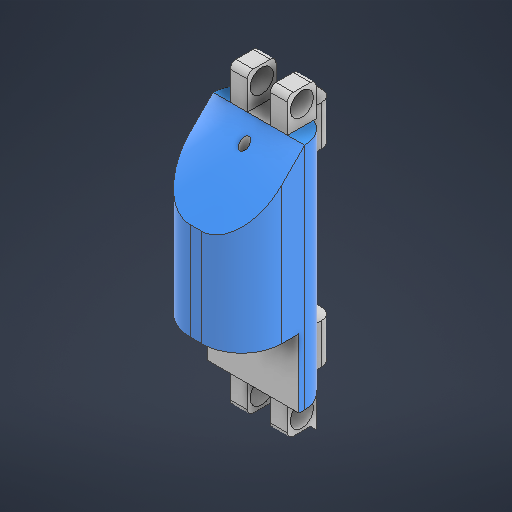
# Autodesk Inventor part: FingerBase
Saved by Autodesk Inventor 2026 (Build 300175050, 175E)
## iProperties
Created: 2026-05-23
Part Number: FingerBase
Material: Generic
Document SubType Name: Modeling
Designer: SaiAn
Density: 1 g/cm^3
Appearance: Default
Author: SaiAn
Autodesk Inventor part; units mm, degrees
ref_plane "YZ Plane" through (0, 0, 0) normal (1, 0, 0) x (0, 1, 0)
ref_plane "XZ Plane" through (0, 0, 0) normal (0, 1, 0) x (-1, 0, 0)
ref_plane "XY Plane" through (0, 0, 0) normal (0, 0, 1) x (1, 0, 0)
sketch "Sketch2" plane through (0, 0, 0) normal (0, 0, 1) x (1, 0, 0)
  line L0 (0, 0) -> (16, 0)
  line L1 (16, 0) -> (16, 40)
  line L2 (16, 40) -> (0, 40)
  line L3 (0, 40) -> (0, 0)
  dimension "d0" = 16
  dimension "d1" = 40
  constraints: 8 end point, 2 parallel, 1 horizontal, 1 perpendicular
  measures "d0" distance of L2.end L1.end
  measures "d1" distance of L1.end L0.end
extrude "Extrusion1" add sketch "Sketch2" along normal blind 16
fillet "Fillet1" radius 7 2 edges at (16, 20, 16) (0, 20, 16)
fillet "Fillet2" radius 5 2 edges at (16, 20, 0) (0, 20, 0)
sketch "Sketch3" plane through (16, 0, 9) normal (1, 0, 0) x (0, 0, -1)
  line L0 (4, 0) -> (4, 40) projected
  line L1 (4, 40) -> (-7, 29)
  line L2 (-7, 0) -> (-7, 40) projected
  line L3 (4, 40) -> (19.5563, 40) construction
  line L4 (-7, 29) -> (-7, 40)
  line L5 (-7, 40) -> (4, 40)
  line L6 (1, 0) -> (12.3137, 0) construction
  line L7 (-7, 8) -> (-7, 0)
  line L8 (1, 0) -> (19.9296, 0) construction
  line L9 (-7, 17.1561) -> (-7, 8)
  point P0 (9, 0)
  dimension "d6" = 135
  constraints: 16 end point, 4 point on line, 3 horizontal, 2 collinear, 1 equal length, 1 perpendicular
  measures "d6" angle of L1 L3
extrude "Extrusion2" cut sketch "Sketch3" against normal through all
sketch "Sketch4" plane through (5, 40, 0) normal (0, 1, 0) x (1, 0, 0)
  line L0 (1, -4.25) -> (5, -0.75) construction
  line L1 (-5, -5) -> (11, -5) projected
  line L2 (1, -5) -> (-2, -5)
  line L3 (-2, -5) -> (-2, 0)
  line L4 (-2, 0) -> (1, 0)
  line L5 (1, 0) -> (1, -5)
  line L6 (5, 0) -> (8, 0)
  line L7 (8, 0) -> (8, -5)
  line L8 (8, -5) -> (5, -5)
  line L9 (5, -5) -> (5, 0)
  point P0 (-5, 0)
  point P1 (-1.888, -0.75)
  point P2 (-1.888, -4.25)
  dimension "d58" = 3
  dimension "d79" = 4
  constraints: 18 end point, 4 parallel, 2 horizontal, 2 perpendicular, 2 point on line
  measures "d58" distance of L3.end L4.end
  measures "d79" distance between parallel lines of L9 L5
extrude "Extrusion3" add sketch "Sketch4" along normal blind 6
sketch "Sketch6" plane through (5, 0, 0) normal (0, -1, 0) x (1, 0, 0)
  line L0 (5, 0) -> (1, 0) projected
  line L1 (8, 0.4174) -> (8, 5) projected
  line L2 (5, 0) -> (8, 0)
  line L3 (8, 0) -> (8, 5)
  line L4 (8, 5) -> (5, 5)
  line L5 (5, 5) -> (5, 0)
  line L6 (-2, 0) -> (-2, 0.4174) projected
  line L7 (-2, 5) -> (1, 5) projected
  line L8 (-2, 0) -> (1, 0)
  line L9 (1, 0) -> (1, 5)
  line L10 (1, 5) -> (-2, 5)
  line L11 (-2, 5) -> (-2, 0)
  point P0 (-5, 0)
  point P1 (-1.888, 0.75)
  point P2 (1, 0.75)
  point P3 (1, 4.25)
  constraints: 16 end point, 4 parallel, 2 horizontal, 2 perpendicular
extrude "Extrusion5" add sketch "Sketch6" along normal blind 6
sketch "Sketch11" plane through (0, 0, 5) normal (-1, 0, 0) x (0, 0, 1)
  line L0 (0, 40) -> (0, 0) projected
  line L1 (11, 0) -> (11, 29) projected
  line L2 (0, 0) -> (11, 0)
  line L3 (11, 0) -> (11, 12)
  line L4 (11, 12) -> (0, 12)
  line L5 (0, 12) -> (0, 0)
  point P0 (-5, 0)
  dimension "d36" = 12
  constraints: 8 end point, 2 parallel, 1 horizontal, 1 perpendicular, 1 point on line
  measures "d36" distance of L3.end L2.end
extrude "Extrusion9" cut sketch "Sketch11" against normal through all
sketch "Sketch12" plane through (0, 0, 0) normal (0, 0, -1) x (-1, 0, 0)
  line L0 (-10, 40) -> (-12.888, 40) projected
  line L1 (-11, 40) -> (-9, 40)
  line L2 (-9, 40) -> (-9, 33)
  line L3 (-9, 33) -> (-11, 33)
  line L4 (-11, 33) -> (-11, 40)
  line L5 (-5, 40) -> (-5, 0) projected
  line L6 (-5, 40) -> (-7, 40)
  line L7 (-7, 40) -> (-7, 33)
  line L8 (-7, 33) -> (-5, 33)
  line L9 (-5, 33) -> (-5, 40)
  line L10 (-12.888, 0) -> (-10, 0) projected
  line L11 (-11, 0) -> (-9, 0)
  line L12 (-9, 0) -> (-9, 7)
  line L13 (-9, 7) -> (-11, 7)
  line L14 (-11, 7) -> (-11, 0)
  line L15 (-5, 0) -> (-7, 0)
  line L16 (-7, 0) -> (-7, 7)
  line L17 (-7, 7) -> (-5, 7)
  line L18 (-5, 7) -> (-5, 0)
  point P0 (0, 0)
  point P1 (-5, 0)
  dimension "d39" = 2
  dimension "d40" = 7
  dimension "d41" = 2
  dimension "d42" = 7
  dimension "d43" = 2
  dimension "d44" = 7
  dimension "d45" = 2
  dimension "d46" = 7
  constraints: 32 end point, 8 parallel, 5 point on line, 4 horizontal, 4 perpendicular
  measures "d39" distance of L2.end L3.end
  measures "d40" distance of L1.end L2.end
  measures "d41" distance of L8.end L7.end
  measures "d42" distance of L7.end L6.end
  measures "d43" distance of L13.end L12.end
  measures "d44" distance of L12.end L11.end
  measures "d45" distance of L16.end L17.end
  measures "d46" distance of L15.end L16.end
extrude "Extrusion10" add sketch "Sketch12" along normal blind 3
sketch "Sketch13" plane through (0, 0, -3) normal (0, 0, -1) x (-1, 0, 0)
  line L0 (-16, 40) -> (-13, 40) projected
  line L1 (-11, 40) -> (-10, 40) projected
  line L2 (-5, 40) -> (-5, 33) projected
  line L3 (-11, 40) -> (-5, 40)
  line L4 (-5, 40) -> (-5, 33)
  line L5 (-5, 33) -> (-11, 33)
  line L6 (-11, 33) -> (-11, 40)
  line L7 (-11, 7) -> (-11, 33) projected
  line L8 (-3, 0) -> (-5, 0) projected
  line L9 (-11, 7) -> (-5, 7)
  line L10 (-5, 7) -> (-5, 0)
  line L11 (-5, 0) -> (-11, 0)
  line L12 (-11, 0) -> (-11, 7)
  point P0 (0, 0)
  constraints: 16 end point, 4 parallel, 2 horizontal, 2 perpendicular
extrude "Extrusion11" add sketch "Sketch13" along normal blind 2
sketch "Sketch14" plane through (0, 12, 5) normal (0, -1, 0) x (1, 0, 0)
  circle A0 centre (8, 2.5) radius 0.75
  line L0 (16, 0) -> (0, 0) projected
  line L1 (16, 4) -> (16, 0) projected
  point P0 (0, -5)
  point P1 (16, 2)
  dimension "d52" = 1.5
  dimension "d55" = 2.5
  dimension "d56" = 8
  constraints: 1 centre point, 1 midpoint
  measures "d52" diameter of A0
  measures "d55" distance from line of A0.centre L0
  measures "d56" horizontal distance of point (16, 2) A0.centre
extrude "Extrusion12" cut sketch "Sketch14" against normal through all
fillet "Fillet5" radius 2 4 edges at (11, 3.5, -5) (5, 3.5, -5) (11, 36.5, -5) (5, 36.5, -5)
sketch "Sketch15" plane through (13, 40, 0.4174) normal (1, 0, 0) x (0, 0, -1)
  circle A0 centre (-2.0826, 3.5) radius 2.025
  line L0 (0.4174, 0) -> (0.4174, 6) projected
  line L1 (-4.5826, 6) -> (0.4174, 6) projected
  point P0 (0.4174, -40)
  point P1 (0.4174, 3)
  dimension "d60" = 4.05
  dimension "d61" = 2.5
  dimension "d62" = 2.5
  constraints: 1 centre point, 1 midpoint
  measures "d60" diameter of A0
  measures "d61" horizontal distance of point (0.417, 3) A0.centre
  measures "d62" distance from line of L1 A0.centre
extrude "Extrusion13" cut sketch "Sketch15" against normal through all
fillet "Fillet6" radius 1 4 edges at (11.5, 46, 0) (11.5, 46, 5) (4.5, 46, 0) (4.5, 46, 5)
sketch "Sketch16" plane through (13, 0, 0.4174) normal (1, 0, 0) x (0, 0, -1)
  circle A0 centre (-2.0826, -3.5) radius 2.025
  line L0 (0.4174, 0) -> (0.4174, -6) projected
  line L1 (0.4174, -6) -> (-4.5826, -6) projected
  dimension "d66" = 4.05
  dimension "d67" = 2.5
  dimension "d68" = 2.5
  constraints: 1 centre point
  measures "d66" diameter of A0
  measures "d67" distance from line of L0 A0.centre
  measures "d68" distance from line of L1 A0.centre
extrude "Extrusion14" cut sketch "Sketch16" against normal through all
fillet "Fillet7" radius 1 2 edges at (4.5, -6, 5) (11.5, -6, 5)
sketch "Sketch17" plane through (5, -6, 0) normal (0, -1, 0) x (1, 0, 0)
  line L0 (8, 0) -> (8, 0.4174) projected
  line L1 (5, 0) -> (5, 5) projected
  line L2 (8, 0) -> (5, 0)
  line L3 (5, 0) -> (5, 1)
  line L4 (5, 1) -> (8, 1)
  line L5 (8, 1) -> (8, 0)
  line L6 (-2, 0) -> (1, 0) projected
  line L7 (-2, 0) -> (1, 0)
  line L8 (1, 0) -> (1, 1)
  line L9 (1, 1) -> (-2, 1)
  line L10 (-2, 1) -> (-2, 0)
  point P0 (-5, 0)
  dimension "d72" = 1
  constraints: 16 end point, 4 parallel, 2 horizontal, 2 perpendicular, 2 point on line
  measures "d72" distance of L2.end L3.end
extrude "Extrusion15" add sketch "Sketch17" along normal blind 1
sketch "Sketch18" plane through (13, 0, 0.4174) normal (1, 0, 0) x (0, 0, -1)
  line L0 (-3.5826, -6) -> (-0.5826, -6) projected
  line L1 (0.4174, 0) -> (0.4174, -7) projected
  line L2 (-0.5826, -6) -> (0.4174, -7)
  line L3 (0.4174, -7) -> (-0.5826, -7)
  line L4 (-0.5826, -7) -> (-0.5826, -6)
  constraints: 6 end point, 2 perpendicular
extrude "Extrusion16" cut sketch "Sketch18" against normal through all
sketch "Sketch19" plane through (6, 0, 5) normal (0, 0, 1) x (-1, 0, 0)
  line L0 (-10, -12) -> (-10, -36) projected
  line L1 (-3, 0) -> (6, 0) projected
  line L2 (-10, -12) -> (6, -12)
  line L3 (6, -12) -> (6, 0)
  line L4 (6, 0) -> (-10, 0)
  line L5 (-10, 0) -> (-10, -12)
  constraints: 8 end point, 2 parallel, 1 horizontal, 1 perpendicular
extrude "Extrusion17" add sketch "Sketch19" along normal blind 1
body "Solid1"
